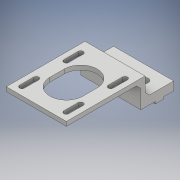
# Autodesk Inventor part: Estrutura - Suporte Z Motor v2
Saved by Autodesk Inventor 2017 (Build 210142000, 142)
## iProperties
Created: 2020-08-02
Part Number: Estrutura - Suporte Z Motor v2
Material: Generic
Document SubType Name: Modeling
Designer: ale
Density: 1 g/cm^3
Appearance: Default
Author: ale
Autodesk Inventor part; units mm, degrees
ref_plane "YZ Plane" through (0, 0, 0) normal (1, 0, 0) x (0, 1, 0)
ref_plane "XZ Plane" through (0, 0, 0) normal (0, 1, 0) x (-1, 0, 0)
ref_plane "XY Plane" through (0, 0, 0) normal (0, 0, 1) x (1, 0, 0)
sketch "Sketch1" plane through (0, 0, 0) normal (0, 0, 1) x (1, 0, 0)
  line L0 (-21, 26) -> (21, 26)
  line L1 (21, 26) -> (21, -26)
  line L2 (21, -26) -> (-21, -26)
  line L3 (-21, -26) -> (-21, 26)
  line L4 (-21, 26) -> (21, -26) construction
  line L5 (21, 26) -> (-21, -26) construction
  line L6 (-15.5, 20.5) -> (15.5, -20.5) construction
  line L7 (15.5, 20.5) -> (-15.5, -20.5) construction
  line L8 (-11.5, -5) -> (-11.5, 5)
  line L9 (11.5, -5) -> (11.5, 5)
  arc A0 (4.507, 5.58) -> (4.2877, 5.6708) centre (0, -5) ccw
  arc A1 (-4.2877, 5.6708) -> (-4.507, 5.58) centre (0, -5) ccw
  arc A2 (-11.5, -5) -> (11.5, -5) centre (0, -5) ccw
  arc A3 (-4.507, -5.58) -> (-4.2877, -5.6708) centre (0, 5) ccw
  arc A4 (4.2877, -5.6708) -> (4.507, -5.58) centre (0, 5) ccw
  arc A5 (11.5, 5) -> (-11.5, 5) centre (0, 5) ccw
  line L10 (-15.5, -20.5) -> (-15.5, -10.5)
  arc A6 (-13.75, -10.5) -> (-17.25, -10.5) centre (-15.5, -10.5) ccw
  line L11 (-13.75, -20.5) -> (-13.75, -10.5)
  line L12 (-17.25, -10.5) -> (-17.25, -20.5)
  arc A7 (-17.25, -20.5) -> (-13.75, -20.5) centre (-15.5, -20.5) ccw
  arc A8 (17.25, -10.5) -> (13.75, -10.5) centre (15.5, -10.5) ccw
  line L13 (17.25, -20.5) -> (17.25, -10.5)
  line L14 (13.75, -10.5) -> (13.75, -20.5)
  arc A9 (13.75, -20.5) -> (17.25, -20.5) centre (15.5, -20.5) ccw
  arc A10 (-13.75, 20.5) -> (-17.25, 20.5) centre (-15.5, 20.5) ccw
  line L15 (-13.75, 10.5) -> (-13.75, 20.5)
  line L16 (-17.25, 20.5) -> (-17.25, 10.5)
  arc A11 (-17.25, 10.5) -> (-13.75, 10.5) centre (-15.5, 10.5) ccw
  arc A12 (17.25, 20.5) -> (13.75, 20.5) centre (15.5, 20.5) ccw
  line L17 (17.25, 10.5) -> (17.25, 20.5)
  line L18 (13.75, 20.5) -> (13.75, 10.5)
  arc A13 (13.75, 10.5) -> (17.25, 10.5) centre (15.5, 10.5) ccw
  point P0 (0, 0)
  dimension "d0" = 42
  dimension "d1" = 52
  dimension "d2" = 31
  dimension "d3" = 41
  dimension "d9" = 5
  dimension "d10" = 5
  dimension "d12" = 10
  dimension "d13" = 3.5
  dimension "d14" = 3.5
  dimension "d15" = 3.5
  dimension "d16" = 3.5
  dimension "d17" = 20.5
  dimension "d18" = 20.5
  dimension "d19" = 20.5
  dimension "d20" = 20.5
  constraints: 38 end point, 28 point on circle, 15 tangent, 14 centre point, 8 point on line, 4 midpoint, 3 parallel, 2 coincident, 1 horizontal, 1 perpendicular
  measures "d0" distance of L1.end L2.end
  measures "d1" distance of L0.end L1.end
  measures "d2" distance of L6.end L7.end
  measures "d3" distance of L7.start L6.end
  measures "d9" distance of point (0, 0) A3.centre
  measures "d10" distance of A0.centre point (0, 0)
  measures "d12" distance of L10.start L10.end
  measures "d13" diameter of A6
  measures "d14" diameter of A8
  measures "d15" diameter of A10
  measures "d16" diameter of A12
  measures "d17" vertical distance of point (0, 0) L6.start
  measures "d18" vertical distance of L7.end point (0, 0)
  measures "d19" vertical distance of L6.end point (0, 0)
  measures "d20" vertical distance of L7.start point (0, 0)
extrude "Extrusion1" add sketch "Sketch1" along normal blind 3
sketch "Sketch2" plane through (-21, 26, 0) normal (0, 1, 0) x (1, 0, 0)
  line L0 (42, -3) -> (0, -3) projected
  line L1 (0, -3) -> (42, -3)
  line L2 (42, -3) -> (42, 10)
  line L3 (42, 10) -> (0, 10)
  line L4 (0, 10) -> (0, -3)
  point P0 (21, 0)
  dimension "d23" = 13
  constraints: 8 end point, 2 parallel, 1 horizontal, 1 perpendicular
  measures "d23" distance of L2.end L1.end
extrude "Extrusion2" add sketch "Sketch2" along normal blind 3
sketch "Sketch3" plane through (21, 26, -10) normal (0, 0, -1) x (-1, 0, 0)
  line L0 (42, 0) -> (0, 0) projected
  line L1 (42, 0) -> (0, 0)
  line L2 (0, 0) -> (0, 23)
  line L3 (0, 23) -> (42, 23)
  line L4 (42, 23) -> (42, 0)
  point P0 (21, -26)
  dimension "d26" = 23
  constraints: 8 end point, 2 parallel, 1 horizontal, 1 perpendicular
  measures "d26" distance of L1.end L2.end
extrude "Extrusion3" add sketch "Sketch3" along normal blind 6
sketch "Sketch6" plane through (21, 26, -10) normal (0, 0, 1) x (1, 0, 0)
  point P0 (-21, -26)
  point P1 (-10.5, 13)
  point P2 (-31.5, 13)
sketch "Sketch7" plane through (21, 26, -16) normal (0, 0, -1) x (-1, 0, 0)
  circle A0 centre (31.5, 13) radius 2.75 projected
  circle A1 centre (10.5, 13) radius 2.75 projected
  line L0 (42, 10) -> (0, 10)
  line L1 (42, 16) -> (0, 16)
  line L2 (42, 0) -> (42, 23) projected
  line L3 (42, 0) -> (42, 23)
  line L4 (0, 0) -> (42, 0) projected
  line L5 (0, 3) -> (0, 23) projected
  line L6 (0, 0) -> (0, 23)
  point P0 (21, -26)
  constraints: 8 end point, 4 point on line, 2 vertical
extrude "Extrusion4" add sketch "Sketch7" along normal blind 1.5 contours L0 L5 L1 L2
sketch "Sketch8" plane through (21, 26, -17.5) normal (0, 0, -1) x (-1, 0, 0)
  circle A0 centre (31.5, 13) radius 2.75 projected
  circle A1 centre (10.5, 13) radius 2.75 projected
  point P0 (21, -26)
  constraints: 2 coincident
hole "Hole2" at (-10.5, 39, -17.5) at (10.5, 39, -17.5) direction (0, 0, 1) diameter 5.5 end through all counterbore diameter 10 counterbore depth 1.5
chamfer "Chamfer2" distance 3 angle 45 2 edges at (0, 26, 0) (0, 29, -10)
body "Solid1"
